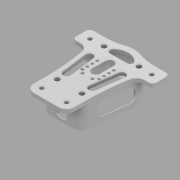
# Autodesk Inventor part: Arm - mounting bottom
Saved by Autodesk Inventor 2017 (Build 210142000, 142)
## iProperties
Created: 2016-04-07
Part Number: Arm - mounting bottom
Material: Generic
Document SubType Name: Modeling
Designer: Ali
Density: 1 g/cm^3
Appearance: Default
Author: Ali
Autodesk Inventor part; units mm, degrees
ref_plane "XZ Plane" through (0, 0, 0) normal (0, 1, 0) x (-1, 0, 0)
sketch "Sketch1" plane through (0, 0, 0) normal (0, 0, 1) x (1, 0, 0)
  circle A0 centre (8.018, -62.9011) radius 2.15 construction
  circle A1 centre (16.3016, 21.0861) radius 2.15 construction
  circle A2 centre (-32.018, -62.9011) radius 2.15 construction
  circle A3 centre (-40.3016, 21.0861) radius 2.15 construction
  arc A4 (-45.0145, -63.2021) -> (-32.018, -75.9011) centre (-32.018, -62.9011) ccw construction
  line L0 (-32.018, -75.9011) -> (8.018, -75.9011) construction
  arc A5 (8.018, -75.9011) -> (21.0145, -63.2021) centre (8.018, -62.9011) ccw projected
  arc A6 (26.6625, -4.5967) -> (21.0145, -63.2021) centre (424.9844, -72.5593) ccw projected
  arc A7 (26.6625, -4.5967) -> (-50.6625, -4.5967) centre (-12, 2) ccw construction
  arc A8 (-45.0145, -63.2021) -> (-50.6625, -4.5967) centre (-448.9844, -72.5593) ccw construction
  circle A9 centre (-12, 2) radius 21 construction
  line L1 (0.5858, -1.5) -> (2.5, -1.5) construction
  line L2 (0.5858, -1.5) -> (0.5858, 0) construction
  line L3 (0.5858, 0) -> (0, 0) construction
  line L4 (0, 0) -> (0, 8.5) construction
  arc A10 (0, 8.5) -> (-4, 12.5) centre (-4, 8.5) ccw construction
  line L5 (-4, 12.5) -> (-20, 12.5) construction
  arc A11 (-20, 12.5) -> (-24, 8.5) centre (-20, 8.5) ccw construction
  line L6 (-24, 8.5) -> (-24, 0) construction
  line L7 (-24.5858, 0) -> (-24, 0) construction
  line L8 (-24.5858, 0) -> (-24.5858, -1.5) construction
  line L9 (-24.5858, -1.5) -> (-26.5, -1.5) construction
  line L10 (-26.5, -1.7) -> (-26.5, -1.5) construction
  line L11 (-26.5, -1.7) -> (-26.9172, -1.7) construction
  line L12 (-26.9172, -1.7) -> (-26.9172, -7.8) construction
  line L13 (-26.9172, -7.8) -> (-24.5858, -7.8) construction
  line L14 (-24.5858, -7.8) -> (-24.5858, -9.7) construction
  line L15 (-24.5858, -9.7) -> (-26.9172, -9.7) construction
  line L16 (-26.9172, -9.7) -> (-26.9172, -15.8) construction
  line L17 (-26.9172, -15.8) -> (-24.5858, -15.8) construction
  line L18 (-24.5858, -15.8) -> (-24.5858, -17.7) construction
  line L19 (-24.5858, -17.7) -> (-26.9172, -17.7) construction
  line L20 (-26.9172, -17.7) -> (-26.9172, -23.8) construction
  line L21 (-26.9172, -23.8) -> (-24.5858, -23.8) construction
  line L22 (-24.5858, -23.8) -> (-24.5858, -25.7) construction
  line L23 (-24.5858, -25.7) -> (-26.9172, -25.7) construction
  line L24 (-26.9172, -25.7) -> (-26.9172, -31.8) construction
  line L25 (-26.9172, -31.8) -> (-25, -31.8) construction
  line L26 (-25, -31.8) -> (-25, -33.5) construction
  line L27 (-23.5, -33.5) -> (-25, -33.5) construction
  line L28 (-23.5, -33.5) -> (-23.5, -35) construction
  line L29 (-23.05, -35) -> (-23.5, -35) construction
  line L30 (-23.05, -35) -> (-23.05, -35.4172) construction
  line L31 (-23.05, -35.4172) -> (-16.95, -35.4172) construction
  line L32 (-16.95, -35.4172) -> (-16.95, -32.9172) construction
  line L33 (-16.95, -32.9172) -> (-7.05, -32.9172) construction
  line L34 (-7.05, -32.9172) -> (-7.05, -35.4172) construction
  line L35 (-7.05, -35.4172) -> (-0.95, -35.4172) construction
  line L36 (-0.95, -35.4172) -> (-0.95, -35) construction
  line L37 (-0.95, -35) -> (-0.5, -35) construction
  line L38 (-0.5, -33.5) -> (-0.5, -35) construction
  line L39 (-0.5, -33.5) -> (1, -33.5) construction
  line L40 (1, -31.8) -> (1, -33.5) construction
  line L41 (1, -31.8) -> (2.9172, -31.8) construction
  line L42 (2.9172, -31.8) -> (2.9172, -25.7) construction
  line L43 (2.9172, -25.7) -> (0.5858, -25.7) construction
  line L44 (0.5858, -25.7) -> (0.5858, -23.8) construction
  line L45 (0.5858, -23.8) -> (2.9172, -23.8) construction
  line L46 (2.9172, -23.8) -> (2.9172, -17.7) construction
  line L47 (2.9172, -17.7) -> (0.5858, -17.7) construction
  line L48 (0.5858, -17.7) -> (0.5858, -15.8) construction
  line L49 (0.5858, -15.8) -> (2.9172, -15.8) construction
  line L50 (2.9172, -15.8) -> (2.9172, -9.7) construction
  line L51 (2.9172, -9.7) -> (0.5858, -9.7) construction
  line L52 (0.5858, -9.7) -> (0.5858, -7.8) construction
  line L53 (0.5858, -7.8) -> (2.9172, -7.8) construction
  line L54 (2.9172, -7.8) -> (2.9172, -1.7) construction
  line L55 (2.9172, -1.7) -> (2.5, -1.7) construction
  line L56 (2.5, -1.7) -> (2.5, -1.5) construction
  line L57 (-26, -2.5) -> (-25, -2.5) construction
  line L58 (-25, -2.5) -> (-25, -3.6044) construction
  arc A12 (-25, -5.8956) -> (-25, -3.6044) centre (-25.5, -4.75) ccw construction
  line L59 (-25, -5.8956) -> (-25, -7) construction
  line L60 (-25, -7) -> (-26, -7) construction
  line L61 (-26, -7) -> (-26, -5.8956) construction
  arc A13 (-26, -3.6044) -> (-26, -5.8956) centre (-25.5, -4.75) ccw construction
  line L62 (-26, -3.6044) -> (-26, -2.5) construction
  line L63 (-26, -10.5) -> (-25, -10.5) construction
  line L64 (-25, -10.5) -> (-25, -11.6044) construction
  arc A14 (-25, -13.8956) -> (-25, -11.6044) centre (-25.5, -12.75) ccw construction
  line L65 (-25, -13.8956) -> (-25, -15) construction
  line L66 (-25, -15) -> (-26, -15) construction
  line L67 (-26, -15) -> (-26, -13.8956) construction
  arc A15 (-26, -11.6044) -> (-26, -13.8956) centre (-25.5, -12.75) ccw construction
  line L68 (-26, -11.6044) -> (-26, -10.5) construction
  line L69 (-26, -18.5) -> (-25, -18.5) construction
  line L70 (-25, -18.5) -> (-25, -19.6044) construction
  arc A16 (-25, -21.8956) -> (-25, -19.6044) centre (-25.5, -20.75) ccw construction
  line L71 (-25, -21.8956) -> (-25, -23) construction
  line L72 (-25, -23) -> (-26, -23) construction
  line L73 (-26, -23) -> (-26, -21.8956) construction
  arc A17 (-26, -19.6044) -> (-26, -21.8956) centre (-25.5, -20.75) ccw construction
  line L74 (-26, -19.6044) -> (-26, -18.5) construction
  line L75 (-26, -26.5) -> (-25, -26.5) construction
  line L76 (-25, -26.5) -> (-25, -27.6044) construction
  arc A18 (-25, -29.8956) -> (-25, -27.6044) centre (-25.5, -28.75) ccw construction
  line L77 (-25, -29.8956) -> (-25, -31.0635) construction
  line L78 (-25, -31.0635) -> (-26, -31.0635) construction
  line L79 (-26, -31.0635) -> (-26, -29.8956) construction
  arc A19 (-26, -27.6044) -> (-26, -29.8956) centre (-25.5, -28.75) ccw construction
  line L80 (-26, -27.6044) -> (-26, -26.5) construction
  line L81 (-2, -8.8) -> (-2, 8.5) construction
  line L82 (-2, -8.8) -> (-1.95, -8.8) construction
  arc A20 (-1.55, -9.2) -> (-1.95, -8.8) centre (-1.95, -9.2) ccw construction
  line L83 (-1.55, -9.2) -> (-1.55, -17.8) construction
  arc A21 (-1.95, -18.2) -> (-1.55, -17.8) centre (-1.95, -17.8) ccw construction
  line L84 (-1.95, -18.2) -> (-2, -18.2) construction
  line L85 (-2, -30.25) -> (-2, -18.2) construction
  arc A22 (-2.25, -30.5) -> (-2, -30.25) centre (-2.25, -30.25) ccw construction
  line L86 (-21.75, -30.5) -> (-2.25, -30.5) construction
  arc A23 (-22, -30.25) -> (-21.75, -30.5) centre (-21.75, -30.25) ccw construction
  line L87 (-22, -18.2) -> (-22, -30.25) construction
  line L88 (-22, -18.2) -> (-22.05, -18.2) construction
  arc A24 (-22.45, -17.8) -> (-22.05, -18.2) centre (-22.05, -17.8) ccw construction
  line L89 (-22.45, -17.8) -> (-22.45, -9.2) construction
  arc A25 (-22.05, -8.8) -> (-22.45, -9.2) centre (-22.05, -9.2) ccw construction
  line L90 (-22.05, -8.8) -> (-22, -8.8) construction
  line L91 (-22, 8.5) -> (-22, -8.8) construction
  arc A26 (-20, 10.5) -> (-22, 8.5) centre (-20, 8.5) ccw construction
  line L92 (-14, 10.5) -> (-20, 10.5) construction
  line L93 (-10, 10.5) -> (-14, 10.5) construction
  line L94 (-4, 10.5) -> (-10, 10.5) construction
  arc A27 (-2, 8.5) -> (-4, 10.5) centre (-4, 8.5) ccw construction
  line L95 (2, -26.5) -> (1, -26.5) construction
  line L96 (2, -27.6044) -> (2, -26.5) construction
  arc A28 (2, -29.8956) -> (2, -27.6044) centre (1.5, -28.75) ccw construction
  line L97 (2, -31.0635) -> (2, -29.8956) construction
  line L98 (1, -31.0635) -> (2, -31.0635) construction
  line L99 (1, -29.8956) -> (1, -31.0635) construction
  arc A29 (1, -27.6044) -> (1, -29.8956) centre (1.5, -28.75) ccw construction
  line L100 (1, -26.5) -> (1, -27.6044) construction
  line L101 (2, -18.5) -> (1, -18.5) construction
  line L102 (2, -19.6044) -> (2, -18.5) construction
  arc A30 (2, -21.8956) -> (2, -19.6044) centre (1.5, -20.75) ccw construction
  line L103 (2, -23) -> (2, -21.8956) construction
  line L104 (1, -23) -> (2, -23) construction
  line L105 (1, -21.8956) -> (1, -23) construction
  arc A31 (1, -19.6044) -> (1, -21.8956) centre (1.5, -20.75) ccw construction
  line L106 (1, -18.5) -> (1, -19.6044) construction
  line L107 (2, -10.5) -> (1, -10.5) construction
  line L108 (2, -11.6044) -> (2, -10.5) construction
  arc A32 (2, -13.8956) -> (2, -11.6044) centre (1.5, -12.75) ccw construction
  line L109 (2, -15) -> (2, -13.8956) construction
  line L110 (1, -15) -> (2, -15) construction
  line L111 (1, -13.8956) -> (1, -15) construction
  arc A33 (1, -11.6044) -> (1, -13.8956) centre (1.5, -12.75) ccw construction
  line L112 (1, -10.5) -> (1, -11.6044) construction
  line L113 (2, -2.5) -> (1, -2.5) construction
  line L114 (2, -3.6044) -> (2, -2.5) construction
  arc A34 (2, -5.8956) -> (2, -3.6044) centre (1.5, -4.75) ccw construction
  line L115 (2, -7) -> (2, -5.8956) construction
  line L116 (1, -7) -> (2, -7) construction
  line L117 (1, -5.8956) -> (1, -7) construction
  arc A35 (1, -3.6044) -> (1, -5.8956) centre (1.5, -4.75) ccw construction
  line L118 (1, -2.5) -> (1, -3.6044) construction
  line L119 (-6.3135, -34.5) -> (-5.1456, -34.5) construction
  line L120 (-6.3135, -33.5) -> (-6.3135, -34.5) construction
  line L121 (-5.1456, -33.5) -> (-6.3135, -33.5) construction
  arc A36 (-2.8544, -33.5) -> (-5.1456, -33.5) centre (-4, -34) ccw construction
  line L122 (-1.6865, -33.5) -> (-2.8544, -33.5) construction
  line L123 (-1.6865, -34.5) -> (-1.6865, -33.5) construction
  line L124 (-2.8544, -34.5) -> (-1.6865, -34.5) construction
  arc A37 (-5.1456, -34.5) -> (-2.8544, -34.5) centre (-4, -34) ccw construction
  line L125 (-17.6865, -33.5) -> (-17.6865, -34.5) construction
  line L126 (-17.6865, -34.5) -> (-18.8544, -34.5) construction
  arc A38 (-21.1456, -34.5) -> (-18.8544, -34.5) centre (-20, -34) ccw construction
  line L127 (-21.1456, -34.5) -> (-22.3135, -34.5) construction
  line L128 (-22.3135, -34.5) -> (-22.3135, -33.5) construction
  line L129 (-22.3135, -33.5) -> (-21.1456, -33.5) construction
  arc A39 (-18.8544, -33.5) -> (-21.1456, -33.5) centre (-20, -34) ccw construction
  line L130 (-18.8544, -33.5) -> (-17.6865, -33.5) construction
  line L131 (-12, -83.0246) -> (-12, 52.1033) construction
  line L132 (-1.5, 12) -> (-12, 12)
  line L133 (-1.5, -31) -> (-12, -31)
  line L134 (-1.5, -31) -> (-1.5, 12)
  line L135 (8.018, -75.9011) -> (-12, -75.9011)
  arc A40 (26.6625, -4.5967) -> (-12, 41.2213) centre (-12, 2) ccw
  arc A41 (-45.0145, -63.2021) -> (-32.018, -75.9011) centre (-32.018, -62.9011) ccw
  arc A42 (-45.0145, -63.2021) -> (-50.6625, -4.5967) centre (-448.9844, -72.5593) ccw
  line L136 (-32.018, -75.9011) -> (-12, -75.9011)
  arc A43 (-12, 41.2213) -> (-50.6625, -4.5967) centre (-12, 2) ccw
  line L137 (-22.5, 12) -> (-12, 12)
  line L138 (-22.5, -31) -> (-12, -31)
  line L139 (-22.5, -31) -> (-22.5, 12)
  dimension "d2" = 21
  dimension "d3" = 10
  dimension "d4" = 33
  constraints: 18 end point, 4 point on circle, 4 point on line, 4 symmetric about line, 2 centre point, 2 perpendicular, 2 vertical, 1 coincident, 1 midpoint, 3 other
  measures "d2" diameter of L134 L131
  measures "d3" distance from line of L132 A7.centre
  measures "d4" distance from line of L133 A7.centre
extrude "Extrusion1" add sketch "Sketch1" along normal blind 5
sketch "Sketch2" plane through (0, 0, 0) normal (0, 0, -1) x (-1, 0, 0)
  line L0 (32.018, -75.9011) -> (-8.018, -75.9011) projected
  arc A0 (32.018, -75.9011) -> (45.0145, -63.2021) centre (32.018, -62.9011) ccw projected
  arc A1 (50.6625, -4.5967) -> (45.0145, -63.2021) centre (448.9844, -72.5593) ccw projected
  arc A2 (50.6625, -4.5967) -> (-26.6625, -4.5967) centre (12, 2) ccw projected
  arc A3 (-21.0145, -63.2021) -> (-26.6625, -4.5967) centre (-424.9844, -72.5593) ccw projected
  arc A4 (-21.0145, -63.2021) -> (-8.018, -75.9011) centre (-8.018, -62.9011) ccw projected
  arc A5 (49.6768, -4.4285) -> (44.0148, -63.179) centre (448.9844, -72.5593) ccw
  line L1 (32.018, -74.9011) -> (-8.018, -74.9011)
  arc A6 (-20.0148, -63.179) -> (-25.6768, -4.4285) centre (-424.9844, -72.5593) ccw
  circle A7 centre (40.3016, 21.0861) radius 2.15 projected
  circle A8 centre (-16.3016, 21.0861) radius 2.15 projected
  circle A9 centre (-8.018, -62.9011) radius 2.15 projected
  circle A10 centre (32.018, -62.9011) radius 2.15 projected
  line L2 (12, 2) -> (40.3016, 21.0861) construction
  line L3 (40.3016, 21.0861) -> (56.7899, 32.2056) construction
  arc A11 (36.9468, 26.0606) -> (43.6563, 16.1116) centre (40.3016, 21.0861) ccw
  line L4 (43.6563, 16.1116) -> (46.6505, 18.1309)
  line L5 (39.9411, 28.0799) -> (36.9468, 26.0606)
  arc A12 (49.6768, -4.4285) -> (46.6505, 18.1309) centre (12, 2) ccw
  line L6 (12, 58.4423) -> (12, -105.8991)
  arc A13 (-19.6563, 16.1116) -> (-12.9468, 26.0606) centre (-16.3016, 21.0861) ccw
  line L7 (-19.6563, 16.1116) -> (-22.6505, 18.1309)
  line L8 (-15.9411, 28.0799) -> (-12.9468, 26.0606)
  arc A14 (39.9411, 28.0799) -> (-15.9411, 28.0799) centre (12, 2) ccw
  arc A15 (-22.6505, 18.1309) -> (-25.6768, -4.4285) centre (12, 2) ccw
  arc A16 (36.8978, -65.7489) -> (34.7521, -67.8455) centre (32.018, -62.9011) ccw
  line L9 (32.018, -62.9011) -> (40.4045, -71.4841) construction
  line L10 (34.7521, -67.8455) -> (39.3316, -72.5324)
  line L11 (36.8978, -65.7489) -> (41.4773, -70.4357)
  arc A17 (32.018, -74.9011) -> (39.2658, -72.465) centre (32.018, -62.9011) ccw
  arc A18 (41.4116, -70.3684) -> (44.0148, -63.179) centre (32.018, -62.9011) ccw
  arc A19 (-10.7521, -67.8455) -> (-12.8978, -65.7489) centre (-8.018, -62.9011) ccw
  line L12 (-10.7521, -67.8455) -> (-15.3316, -72.5324)
  line L13 (-12.8978, -65.7489) -> (-17.4773, -70.4357)
  arc A20 (-20.0148, -63.179) -> (-17.4116, -70.3684) centre (-8.018, -62.9011) ccw
  arc A21 (-15.2658, -72.465) -> (-8.018, -74.9011) centre (-8.018, -62.9011) ccw
  point P0 (0, 0)
  point P1 (48.5457, 26.6459)
  dimension "d9" = 6
  dimension "d10" = 3.5
  dimension "d11" = 1.5
  constraints: 28 end point, 26 point on circle, 13 centre point, 12 symmetric about line, 5 point on line, 2 parallel, 2 tangent, 1 midpoint, 1 vertical, 2 other
  measures "d9" radius of A11
  measures "d10" radial gap between concentric circles of A10 A16
  measures "d11" distance between parallel lines of L9 L10
ref_plane "Work Plane1" through (-51.2213, -75.9011, -38) normal (0, 0, 1) x (1, 0, 0)
extrude "Extrusion2" add sketch "Sketch2" along normal up to surface (38 mm away) contours L0 L6 L1 A17 L10 A16 L11 A18 A5 A12 L4 A11 L5 A14 A2 A1 A0 | L0 A4 A3 A2 L6 A14 L8 A13 L7 A15 A6 A20 L13 A19 L12 A21 L1
sketch "Sketch4" plane through (-32.018, -75.9011, 5) normal (0, -1, 0) x (1, 0, 0)
  line L0 (22.7813, -17.9259) -> (17.2547, -17.9259)
  line L1 (11.2547, -23.9259) -> (11.2547, -32.7215)
  line L2 (17.2547, -38.7215) -> (22.7813, -38.7215)
  line L3 (28.7813, -32.7215) -> (28.7813, -23.9259)
  line L4 (28.7813, -17.9259) -> (11.2547, -38.7215) construction
  line L5 (11.2547, -17.9259) -> (28.7813, -38.7215) construction
  arc A0 (22.7813, -38.7215) -> (28.7813, -32.7215) centre (22.7813, -32.7215) ccw
  arc A1 (11.2547, -32.7215) -> (17.2547, -38.7215) centre (17.2547, -32.7215) ccw
  arc A2 (17.2547, -17.9259) -> (11.2547, -23.9259) centre (17.2547, -23.9259) ccw
  arc A3 (28.7813, -23.9259) -> (22.7813, -17.9259) centre (22.7813, -23.9259) ccw
  point P0 (32.018, -5)
  point P1 (20.018, -28.3237)
  dimension "d16" = 6
  constraints: 12 end point, 8 point on circle, 8 point on line, 8 tangent, 4 centre point, 3 equal radius, 2 midpoint, 2 parallel, 1 horizontal, 1 perpendicular, 1 other
  measures "d16" radius of A0
extrude "Extrusion4" cut sketch "Sketch4" against normal up to next
fillet "Fillet1" radius 2 34 edges at (-46.6505, 18.1309, -19) (-39.9411, 28.0799, -19) (-41.4116, -70.3684, -19) (-36.8978, -65.7489, -19) (-39.2658, -72.465, -19) (-34.7521, -67.8455, -19) (-49.8819, 7.0817, 0) (-43.3011, -66.9866, 0) (-45.7743, -33.7005, 0) (-12, 40.2213, 0) (-38.444, 27.0703, 0) (-45.1534, 17.1212, 0) (-35.3271, 17.7314, 0) (-35.8411, -74.2758, 0) (11.8411, -74.2758, 0) (-12, -74.9011, 0) (19.3011, -66.9866, 0) (25.8819, 7.0817, 0) (21.7743, -33.7005, 0) (4.0694, -58.8599, 0) (10.7521, -67.8455, -19) (15.2658, -72.465, -19) (17.4116, -70.3684, -19) (12.8978, -65.7489, -19) (13.0089, -70.1553, 0) (15.1547, -68.0587, 0) (-39.1547, -68.0587, 0) (-37.0089, -70.1553, 0) (15.9411, 28.0799, -19) (21.1534, 17.1212, 0) (14.444, 27.0703, 0) (11.3271, 17.7314, 0) (22.6505, 18.1309, -19) (-28.0694, -58.8599, 0)
sketch "Sketch7" plane through (0, 0, 0) normal (0, 0, -1) x (-1, 0, 0)
  line L0 (1.5, -31) -> (22.5, -31) projected
  line L1 (16.5002, -31) -> (7.5045, -31)
  line L2 (7.5045, -31) -> (7.5045, -53.6732)
  line L3 (7.5045, -53.6732) -> (16.5002, -53.6732)
  line L4 (16.5002, -53.6732) -> (16.5002, -31)
  point P0 (0, 0)
  constraints: 8 end point, 2 parallel, 1 horizontal, 1 perpendicular, 1 point on line
extrude "Extrusion7" cut sketch "Sketch7" against normal blind 3.5
fillet "Fillet3" radius 6 2 edges at (-12.0024, -53.6732, 3.5) (-12.0024, -53.6732, 0)
sketch "Sketch8" plane through (0, 0, 5) normal (0, 0, 1) x (1, 0, 0)
  line L0 (-1.5, 12) -> (-1.5, -31) projected
  line L1 (-1.5, -31) -> (-22.5, -31) projected
  line L2 (-22.5, -31) -> (-22.5, 12) projected
  line L3 (-22.5, 12) -> (-1.5, 12) projected
  point P0 (0, 0)
extrude "Extrusion8" add sketch "Sketch8" against normal blind 1.5
sketch "Sketch10" plane through (0, 0, 5) normal (0, 0, 1) x (1, 0, 0)
  line L0 (-70.7409, 34.4584) -> (-34.0172, 34.4584)
  line L1 (52.7409, 28.4584) -> (52.7409, 12.5917)
  line L2 (46.7409, 6.5917) -> (26.9516, 6.5917)
  line L3 (-76.7409, 12.5917) -> (-76.7409, 20.525)
  line L4 (-12, 67.6046) -> (-12, -83.4161) construction
  line L5 (10.0172, 34.4584) -> (46.7409, 34.4584)
  line L6 (-123.6927, 20.525) -> (99.0882, 20.525) construction
  line L7 (-76.7409, 20.525) -> (-76.7409, 28.4584)
  arc A0 (46.7409, 6.5917) -> (52.7409, 12.5917) centre (46.7409, 12.5917) ccw
  arc A1 (52.7409, 28.4584) -> (46.7409, 34.4584) centre (46.7409, 28.4584) ccw
  arc A2 (-70.7409, 34.4584) -> (-76.7409, 28.4584) centre (-70.7409, 28.4584) ccw
  arc A3 (-76.7409, 12.5917) -> (-70.7409, 6.5917) centre (-70.7409, 12.5917) ccw
  arc A4 (26.9516, 6.5917) -> (10.0172, 34.4584) centre (-12, 2) ccw
  arc A5 (-34.0172, 34.4584) -> (-50.9516, 6.5917) centre (-12, 2) ccw
  line L8 (-50.9516, 6.5917) -> (-70.7409, 6.5917)
  line L9 (-32.018, -100.9245) -> (-12, -100.9245)
  arc A6 (8.018, -100.9245) -> (21.0145, -88.2255) centre (8.018, -87.9245) ccw
  arc A7 (-45.0145, -88.2255) -> (-32.018, -100.9245) centre (-32.018, -87.9245) ccw
  line L10 (-12, -100.9245) -> (8.018, -100.9245)
  line L11 (21.0145, -88.2255) -> (21.0145, -63.2021)
  arc A8 (8.018, -75.9011) -> (21.0145, -63.2021) centre (8.018, -62.9011) ccw projected
  line L12 (-32.018, -75.9011) -> (8.018, -75.9011) projected
  arc A9 (-45.0145, -63.2021) -> (-32.018, -75.9011) centre (-32.018, -62.9011) ccw projected
  line L13 (-45.0145, -88.2255) -> (-45.0145, -63.2021)
  point P0 (0, 0)
  dimension "d30" = 6
  dimension "d31" = 6
  constraints: 26 end point, 18 point on circle, 10 tangent, 8 centre point, 6 parallel, 4 horizontal, 3 point on line, 3 vertical, 2 collinear, 2 equal radius, 2 perpendicular, 1 other
  measures "d30" radius of A0
  measures "d31" radius of A1
extrude "Extrusion9" add sketch "Sketch10" against normal blind 6
fillet "Fillet4" radius 90 2 edges at (-34.0172, 34.4584, 2) (10.0172, 34.4584, 2)
fillet "Fillet5" radius 13.75 2 edges at (26.9516, 6.5917, 2) (-50.9516, 6.5917, 2)
fillet "Fillet6" radius 3 7 edges at (26.6406, -4.7256, -1) (21.6722, 22.112, -1) (-50.6406, -4.7256, -1) (-45.6722, 22.112, -1) (-41.1033, -72.1993, -1) (17.1033, -72.1993, -1) (-12, -75.9011, -1)
sketch "Sketch11" plane through (0, 0, 5) normal (0, 0, 1) x (1, 0, 0)
  arc A0 (40.1743, 6.5917) -> (26.6186, -4.8545) centre (40.1743, -7.1583) ccw projected
  line L0 (46.7409, 6.5917) -> (40.1743, 6.5917) projected
  arc A1 (46.7409, 6.5917) -> (52.7409, 12.5917) centre (46.7409, 12.5917) ccw projected
  line L1 (52.7409, 28.4584) -> (52.7409, 12.5917) projected
  arc A2 (52.7409, 28.4584) -> (46.7409, 34.4584) centre (46.7409, 28.4584) ccw projected
  line L2 (29.2562, 34.4584) -> (46.7409, 34.4584) projected
  arc A3 (0.5221, 39.1686) -> (29.2562, 34.4584) centre (29.2562, 124.4584) ccw projected
  arc A4 (0.5221, 39.1686) -> (-24.5221, 39.1686) centre (-12, 2) ccw projected
  arc A5 (-53.2562, 34.4584) -> (-24.5221, 39.1686) centre (-53.2562, 124.4584) ccw projected
  line L3 (-53.2562, 34.4584) -> (-70.7409, 34.4584) projected
  arc A6 (-70.7409, 34.4584) -> (-76.7409, 28.4584) centre (-70.7409, 28.4584) ccw projected
  line L4 (-76.7409, 28.4584) -> (-76.7409, 12.5917) projected
  arc A7 (-76.7409, 12.5917) -> (-70.7409, 6.5917) centre (-70.7409, 12.5917) ccw projected
  line L5 (-70.7409, 6.5917) -> (-64.1743, 6.5917) projected
  arc A8 (-50.6186, -4.8545) -> (-64.1743, 6.5917) centre (-64.1743, -7.1583) ccw projected
  arc A9 (-45.0145, -63.2021) -> (-50.6186, -4.8545) centre (-448.9844, -72.5593) ccw projected
  line L6 (-45.0145, -63.2021) -> (-45.0145, -88.2255) projected
  arc A10 (-45.0145, -88.2255) -> (-32.018, -100.9245) centre (-32.018, -87.9245) ccw projected
  line L7 (-32.018, -100.9245) -> (8.018, -100.9245) projected
  arc A11 (8.018, -100.9245) -> (21.0145, -88.2255) centre (8.018, -87.9245) ccw projected
  line L8 (21.0145, -88.2255) -> (21.0145, -63.2021) projected
  arc A12 (26.6186, -4.8545) -> (21.0145, -63.2021) centre (424.9844, -72.5593) ccw projected
  line L9 (-12, 2) -> (-12, 28.4584)
  point P0 (0, 0)
  point P1 (38, 20.0755)
  point P2 (-62, 20.0755)
  point P3 (-32.018, -87.9245)
  dimension "d44" = 100
  dimension "d45" = 108
  constraints: 2 end point, 2 symmetric about line, 1 coincident, 1 vertical
  measures "d44" distance of point (-62, 20.076) point (38, 20.076)
  measures "d45" vertical distance of point (-62, 20.076) point (-32.018, -87.924)
hole "Hole1" at (38, 20.0755, 5) at (8.018, -87.9245, 5) at (-62, 20.0755, 5) at (-32.018, -87.9245, 5) direction (0, 0, -1) diameter 6.5 end through all
sketch "Sketch12" plane through (0, 0, 5) normal (0, 0, 1) x (1, 0, 0)
  circle A0 centre (8.018, -62.9011) radius 2.15 projected
  circle A1 centre (-32.018, -62.9011) radius 2.15 projected
  circle A2 centre (-40.3016, 21.0861) radius 2.15 projected
  circle A3 centre (16.3016, 21.0861) radius 2.15 projected
  point P0 (0, 0)
hole "Hole2" at (-32.018, -62.9011, 5) at (8.018, -62.9011, 5) at (-40.3016, 21.0861, 5) at (16.3016, 21.0861, 5) direction (0, 0, -1) diameter 4.5 end through all counterbore diameter 8 counterbore depth 10
chamfer "Chamfer1" distance 1.75 angle 45 4 edges at (-32.018, -60.6511, -5) (-40.3016, 23.3361, -5) (16.3016, 23.3361, -5) (8.018, -60.6511, -5)
sketch "Sketch13" plane through (0, 0, 5) normal (0, 0, 1) x (1, 0, 0)
  line L0 (0.5858, 0) -> (0, 0) projected
  line L1 (0.5858, 0) -> (0.5858, -1.5) projected
  line L2 (0.5858, -1.5) -> (2.5, -1.5) projected
  line L3 (2.5, -1.7) -> (2.5, -1.5) projected
  line L4 (2.5, -1.7) -> (2.9172, -1.7) projected
  line L5 (2.9172, -1.7) -> (2.9172, -7.8) projected
  line L6 (2.9172, -7.8) -> (0.5858, -7.8) projected
  line L7 (0.5858, -7.8) -> (0.5858, -9.7) projected
  line L8 (0.5858, -9.7) -> (2.9172, -9.7) projected
  line L9 (2.9172, -9.7) -> (2.9172, -15.8) projected
  line L10 (2.9172, -15.8) -> (0.5858, -15.8) projected
  line L11 (0.5858, -15.8) -> (0.5858, -17.7) projected
  line L12 (0.5858, -17.7) -> (2.9172, -17.7) projected
  line L13 (2.9172, -17.7) -> (2.9172, -23.8) projected
  line L14 (2.9172, -23.8) -> (0.5858, -23.8) projected
  line L15 (0.5858, -23.8) -> (0.5858, -25.7) projected
  line L16 (0.5858, -25.7) -> (2.9172, -25.7) projected
  line L17 (2.9172, -25.7) -> (2.9172, -31.8) projected
  line L18 (2.9172, -31.8) -> (1, -31.8) projected
  line L19 (1, -31.8) -> (1, -33.5) projected
  line L20 (-0.5, -33.5) -> (1, -33.5) projected
  line L21 (-0.5, -33.5) -> (-0.5, -35) projected
  line L22 (-0.95, -35) -> (-0.5, -35) projected
  line L23 (-0.95, -35) -> (-0.95, -35.4172) projected
  line L24 (-0.95, -35.4172) -> (-7.05, -35.4172) projected
  line L25 (-7.05, -35.4172) -> (-7.05, -32.9172) projected
  line L26 (-7.05, -32.9172) -> (-16.95, -32.9172) projected
  line L27 (-16.95, -32.9172) -> (-16.95, -35.4172) projected
  line L28 (-16.95, -35.4172) -> (-23.05, -35.4172) projected
  line L29 (-23.05, -35.4172) -> (-23.05, -35) projected
  line L30 (-23.05, -35) -> (-23.5, -35) projected
  line L31 (-23.5, -33.5) -> (-23.5, -35) projected
  line L32 (-23.5, -33.5) -> (-25, -33.5) projected
  line L33 (-25, -31.8) -> (-25, -33.5) projected
  line L34 (-25, -31.8) -> (-26.9172, -31.8) projected
  line L35 (-26.9172, -31.8) -> (-26.9172, -25.7) projected
  line L36 (-26.9172, -25.7) -> (-24.5858, -25.7) projected
  line L37 (-24.5858, -25.7) -> (-24.5858, -23.8) projected
  line L38 (-24.5858, -23.8) -> (-26.9172, -23.8) projected
  line L39 (-26.9172, -23.8) -> (-26.9172, -17.7) projected
  line L40 (-26.9172, -17.7) -> (-24.5858, -17.7) projected
  line L41 (-24.5858, -17.7) -> (-24.5858, -15.8) projected
  line L42 (-24.5858, -15.8) -> (-26.9172, -15.8) projected
  line L43 (-26.9172, -15.8) -> (-26.9172, -9.7) projected
  line L44 (-26.9172, -9.7) -> (-24.5858, -9.7) projected
  line L45 (-24.5858, -9.7) -> (-24.5858, -7.8) projected
  line L46 (-24.5858, -7.8) -> (-26.9172, -7.8) projected
  line L47 (-26.9172, -7.8) -> (-26.9172, -1.7) projected
  line L48 (-26.9172, -1.7) -> (-26.5, -1.7) projected
  line L49 (-26.5, -1.7) -> (-26.5, -1.5) projected
  line L50 (-24.5858, -1.5) -> (-26.5, -1.5) projected
  line L51 (-24.5858, -1.5) -> (-24.5858, 0) projected
  line L52 (-24.5858, 0) -> (-24, 0) projected
  line L53 (-24, 0) -> (-24, 8.25) projected
  line L54 (-24, 8.25) -> (-22, 8.25) projected
  line L55 (-22, -27.25) -> (-22, 8.25) projected
  arc A0 (-22, -27.25) -> (-21.9959, -27.2951) centre (-21.75, -27.25) ccw projected
  arc A1 (-21.9959, -27.2951) -> (-18.7951, -30.4959) centre (-21.5, -30) ccw projected
  arc A2 (-18.7951, -30.4959) -> (-18.75, -30.5) centre (-18.75, -30.25) ccw projected
  line L56 (-5.25, -30.5) -> (-18.75, -30.5) projected
  arc A3 (-5.25, -30.5) -> (-5.2049, -30.4959) centre (-5.25, -30.25) ccw projected
  arc A4 (-5.2049, -30.4959) -> (-2.0041, -27.2951) centre (-2.5, -30) ccw projected
  arc A5 (-2.0041, -27.2951) -> (-2, -27.25) centre (-2.25, -27.25) ccw projected
  line L57 (-2, 8.25) -> (-2, -27.25) projected
  line L58 (-2, 8.25) -> (0, 8.25) projected
  line L59 (0, 8.25) -> (0, 0) projected
  line L60 (2, -2.5) -> (1, -2.5) projected
  line L61 (1, -2.5) -> (1, -3.6044) projected
  arc A6 (1, -3.6044) -> (1, -5.8956) centre (1.5, -4.75) ccw projected
  line L62 (1, -5.8956) -> (1, -7) projected
  line L63 (1, -7) -> (2, -7) projected
  line L64 (2, -7) -> (2, -5.8956) projected
  arc A7 (2, -5.8956) -> (2, -3.6044) centre (1.5, -4.75) ccw projected
  line L65 (2, -3.6044) -> (2, -2.5) projected
  line L66 (2, -10.5) -> (1, -10.5) projected
  line L67 (1, -10.5) -> (1, -11.6044) projected
  arc A8 (1, -11.6044) -> (1, -13.8956) centre (1.5, -12.75) ccw projected
  line L68 (1, -13.8956) -> (1, -15) projected
  line L69 (1, -15) -> (2, -15) projected
  line L70 (2, -15) -> (2, -13.8956) projected
  arc A9 (2, -13.8956) -> (2, -11.6044) centre (1.5, -12.75) ccw projected
  line L71 (2, -11.6044) -> (2, -10.5) projected
  line L72 (2, -18.5) -> (1, -18.5) projected
  line L73 (1, -18.5) -> (1, -19.6044) projected
  arc A10 (1, -19.6044) -> (1, -21.8956) centre (1.5, -20.75) ccw projected
  line L74 (1, -21.8956) -> (1, -23) projected
  line L75 (1, -23) -> (2, -23) projected
  line L76 (2, -23) -> (2, -21.8956) projected
  arc A11 (2, -21.8956) -> (2, -19.6044) centre (1.5, -20.75) ccw projected
  line L77 (2, -19.6044) -> (2, -18.5) projected
  line L78 (2, -26.5) -> (1, -26.5) projected
  line L79 (1, -26.5) -> (1, -27.6044) projected
  arc A12 (1, -27.6044) -> (1, -29.8956) centre (1.5, -28.75) ccw projected
  line L80 (1, -29.8956) -> (1, -31.0635) projected
  line L81 (1, -31.0635) -> (2, -31.0635) projected
  line L82 (2, -31.0635) -> (2, -29.8956) projected
  arc A13 (2, -29.8956) -> (2, -27.6044) centre (1.5, -28.75) ccw projected
  line L83 (2, -27.6044) -> (2, -26.5) projected
  line L84 (-26, -18.5) -> (-25, -18.5) projected
  line L85 (-26, -19.6044) -> (-26, -18.5) projected
  arc A14 (-26, -19.6044) -> (-26, -21.8956) centre (-25.5, -20.75) ccw projected
  line L86 (-26, -23) -> (-26, -21.8956) projected
  line L87 (-25, -23) -> (-26, -23) projected
  line L88 (-25, -21.8956) -> (-25, -23) projected
  arc A15 (-25, -21.8956) -> (-25, -19.6044) centre (-25.5, -20.75) ccw projected
  line L89 (-25, -18.5) -> (-25, -19.6044) projected
  line L90 (-26, -10.5) -> (-25, -10.5) projected
  line L91 (-26, -11.6044) -> (-26, -10.5) projected
  arc A16 (-26, -11.6044) -> (-26, -13.8956) centre (-25.5, -12.75) ccw projected
  line L92 (-26, -15) -> (-26, -13.8956) projected
  line L93 (-25, -15) -> (-26, -15) projected
  line L94 (-25, -13.8956) -> (-25, -15) projected
  arc A17 (-25, -13.8956) -> (-25, -11.6044) centre (-25.5, -12.75) ccw projected
  line L95 (-25, -10.5) -> (-25, -11.6044) projected
  line L96 (-26, -2.5) -> (-25, -2.5) projected
  line L97 (-26, -3.6044) -> (-26, -2.5) projected
  arc A18 (-26, -3.6044) -> (-26, -5.8956) centre (-25.5, -4.75) ccw projected
  line L98 (-26, -7) -> (-26, -5.8956) projected
  line L99 (-25, -7) -> (-26, -7) projected
  line L100 (-25, -5.8956) -> (-25, -7) projected
  arc A19 (-25, -5.8956) -> (-25, -3.6044) centre (-25.5, -4.75) ccw projected
  line L101 (-25, -2.5) -> (-25, -3.6044) projected
  line L102 (-26, -26.5) -> (-25, -26.5) projected
  line L103 (-26, -27.6044) -> (-26, -26.5) projected
  arc A20 (-26, -27.6044) -> (-26, -29.8956) centre (-25.5, -28.75) ccw projected
  line L104 (-26, -31.0635) -> (-26, -29.8956) projected
  line L105 (-25, -31.0635) -> (-26, -31.0635) projected
  line L106 (-25, -29.8956) -> (-25, -31.0635) projected
  arc A21 (-25, -29.8956) -> (-25, -27.6044) centre (-25.5, -28.75) ccw projected
  line L107 (-25, -26.5) -> (-25, -27.6044) projected
  line L108 (-17.6865, -34.5) -> (-18.8544, -34.5) projected
  line L109 (-17.6865, -33.5) -> (-17.6865, -34.5) projected
  line L110 (-18.8544, -33.5) -> (-17.6865, -33.5) projected
  arc A22 (-18.8544, -33.5) -> (-21.1456, -33.5) centre (-20, -34) ccw projected
  line L111 (-22.3135, -33.5) -> (-21.1456, -33.5) projected
  line L112 (-22.3135, -34.5) -> (-22.3135, -33.5) projected
  line L113 (-21.1456, -34.5) -> (-22.3135, -34.5) projected
  arc A23 (-21.1456, -34.5) -> (-18.8544, -34.5) centre (-20, -34) ccw projected
  line L114 (-6.3135, -33.5) -> (-6.3135, -34.5) projected
  line L115 (-6.3135, -34.5) -> (-5.1456, -34.5) projected
  arc A24 (-5.1456, -34.5) -> (-2.8544, -34.5) centre (-4, -34) ccw projected
  line L116 (-2.8544, -34.5) -> (-1.6865, -34.5) projected
  line L117 (-1.6865, -34.5) -> (-1.6865, -33.5) projected
  line L118 (-1.6865, -33.5) -> (-2.8544, -33.5) projected
  arc A25 (-2.8544, -33.5) -> (-5.1456, -33.5) centre (-4, -34) ccw projected
  line L119 (-5.1456, -33.5) -> (-6.3135, -33.5) projected
hole "Hole3" at (-4, -34, 5) at (-20, -34, 5) at (-25.5, -28.75, 5) at (-25.5, -20.75, 5) at (-25.5, -12.75, 5) at (-25.5, -4.75, 5) at (1.5, -28.75, 5) at (1.5, -20.75, 5) at (1.5, -12.75, 5) at (1.5, -4.75, 5) direction (0, 0, -1) diameter 2.5 end through all counterbore diameter 4.5 counterbore depth 2.2
chamfer "Chamfer2" distance 1 angle 45 10 edges at (-4, -32.75, 2.8) (1.5, -27.5, 2.8) (1.5, -19.5, 2.8) (1.5, -11.5, 2.8) (1.5, -3.5, 2.8) (-20, -32.75, 2.8) (-25.5, -27.5, 2.8) (-25.5, -19.5, 2.8) (-25.5, -11.5, 2.8) (-25.5, -3.5, 2.8)
ref_plane "Work Plane4" through (-60, 0, 0) normal (-1, 0, 0) x (0, -1, 0)
sketch "Sketch16" plane through (-12, 2, -38) normal (0, 0, -1) x (-1, 0, 0)
  arc A0 (-33.0145, -65.2021) -> (-20.018, -77.9011) centre (-20.018, -64.9011) ccw projected
  arc A1 (-33.0145, -65.2021) -> (-38.6625, -6.5967) centre (-436.9844, -74.5593) ccw projected
  arc A2 (38.6625, -6.5967) -> (-38.6625, -6.5967) centre (0, 0) ccw projected
  arc A3 (38.6625, -6.5967) -> (33.0145, -65.2021) centre (436.9844, -74.5593) ccw projected
  arc A4 (20.018, -77.9011) -> (33.0145, -65.2021) centre (20.018, -64.9011) ccw projected
  line L0 (-20.018, -77.9011) -> (20.018, -77.9011) projected
  arc A5 (-29.0156, -65.1095) -> (-20.018, -73.9011) centre (-20.018, -64.9011) ccw
  arc A6 (-29.0156, -65.1095) -> (-34.7195, -5.9239) centre (-436.9844, -74.5593) ccw
  arc A7 (34.7195, -5.9239) -> (-34.7195, -5.9239) centre (0, 0) ccw
  arc A8 (34.7195, -5.9239) -> (29.0156, -65.1095) centre (436.9844, -74.5593) ccw
  arc A9 (20.018, -73.9011) -> (29.0156, -65.1095) centre (20.018, -64.9011) ccw
  line L1 (20.018, -73.9011) -> (-20.018, -73.9011)
  point P0 (-12, -2)
  dimension "d69" = 4
  constraints: 10 point on circle, 5 centre point, 2 end point, 5 other
  measures "d69" radial gap between concentric circles of A0 A5
extrude "Extrusion10" add sketch "Sketch16" against normal blind 3
chamfer "Chamfer3" distance 3 angle 45 10 edges at (-12, 37.2213, -35) (-46.9395, 6.4461, -35) (-42.7881, -33.4127, -35) (-40.543, -65.7863, -35) (22.9395, 6.4461, -35) (18.7881, -33.4127, -35) (16.543, -65.7863, -35) (-12, -71.9011, -35) (-34.7051, -71.4906, -35) (10.7051, -71.4906, -35)
sketch "Sketch17" plane through (0, 0, 0) normal (0, 0, -1) x (-1, 0, 0)
  circle A0 centre (-1.5, -12.75) radius 1.25 projected
  circle A1 centre (-1.5, -28.75) radius 1.25 projected
  circle A2 centre (25.5, -12.75) radius 1.25 projected
  circle A3 centre (25.5, -28.75) radius 1.25 projected
  circle A4 centre (4, -34) radius 1.25 projected
  circle A5 centre (20, -34) radius 1.25 projected
  circle A6 centre (25.5, -20.75) radius 1.25 projected
  circle A7 centre (25.5, -4.75) radius 1.25 projected
  circle A8 centre (-1.5, -20.75) radius 1.25 projected
  circle A9 centre (-1.5, -4.75) radius 1.25 projected
  line L0 (7.5045, -56.6894) -> (7.5045, -31) projected
  line L1 (7.5045, -31) -> (1.5, -31) projected
  line L2 (1.5, -31) -> (1.5, 12) projected
  line L3 (1.5, 12) -> (22.5, 12) projected
  line L4 (22.5, 12) -> (22.5, -31) projected
  line L5 (22.5, -31) -> (16.5002, -31) projected
  line L6 (16.5002, -56.6894) -> (16.5002, -31) projected
  line L7 (7.5045, -56.6894) -> (16.5002, -56.6894) projected
  arc A10 (-12.0613, -72.0472) -> (-8.018, -72.9011) centre (-8.018, -62.9011) ccw projected
  line L8 (32.018, -72.9011) -> (-8.018, -72.9011) projected
  arc A11 (32.018, -72.9011) -> (36.0613, -72.0472) centre (32.018, -62.9011) ccw projected
  line L9 (34.2686, -70.2125) -> (36.0613, -72.0472) projected
  arc A12 (39.2754, -65.3204) -> (34.2686, -70.2125) centre (32.018, -62.9011) ccw projected
  line L10 (41.068, -67.1551) -> (39.2754, -65.3204) projected
  arc A13 (41.068, -67.1551) -> (42.0153, -63.1327) centre (32.018, -62.9011) ccw projected
  arc A14 (47.7053, -4.0921) -> (42.0153, -63.1327) centre (448.9844, -72.5593) ccw projected
  arc A15 (47.7053, -4.0921) -> (45.7619, 15.1193) centre (12, 2) ccw projected
  line L11 (44.7745, 14.4534) -> (45.7619, 15.1193) projected
  arc A16 (35.8286, 27.7188) -> (44.7745, 14.4534) centre (40.3016, 21.0861) ccw projected
  line L12 (36.8159, 28.3847) -> (35.8286, 27.7188) projected
  arc A17 (36.8159, 28.3847) -> (-12.8159, 28.3847) centre (12, 2) ccw projected
  line L13 (-11.8286, 27.7188) -> (-12.8159, 28.3847) projected
  arc A18 (-20.7745, 14.4534) -> (-11.8286, 27.7188) centre (-16.3016, 21.0861) ccw projected
  line L14 (-21.7619, 15.1193) -> (-20.7745, 14.4534) projected
  arc A19 (-21.7619, 15.1193) -> (-23.7053, -4.0921) centre (12, 2) ccw projected
  arc A20 (-18.0153, -63.1327) -> (-23.7053, -4.0921) centre (-424.9844, -72.5593) ccw projected
  arc A21 (-18.0153, -63.1327) -> (-17.068, -67.1551) centre (-8.018, -62.9011) ccw projected
  line L15 (-15.2754, -65.3204) -> (-17.068, -67.1551) projected
  arc A22 (-10.2686, -70.2125) -> (-15.2754, -65.3204) centre (-8.018, -62.9011) ccw projected
  line L16 (-12.0613, -72.0472) -> (-10.2686, -70.2125) projected
  line L17 (32.5187, -46.656) -> (38.2234, -4.6893) construction
  line L18 (38.4217, -47.4584) -> (44.1264, -5.4917)
  line L19 (32.3204, -3.8868) -> (26.6157, -45.8536)
  arc A23 (26.6157, -45.8536) -> (38.4217, -47.4584) centre (32.5187, -46.656) ccw
  arc A24 (44.1264, -5.4917) -> (32.3204, -3.8868) centre (38.2234, -4.6893) ccw
  line L20 (25.8821, 21.0861) -> (-1.8821, 21.0861) construction
  line L21 (25.8821, 16.1256) -> (-1.8821, 16.1256)
  arc A25 (25.8821, 16.1256) -> (29.4681, 24.5136) centre (25.8821, 21.0861) ccw
  arc A26 (-5.4681, 24.5136) -> (-1.8821, 16.1256) centre (-1.8821, 21.0861) ccw
  line L22 (32.018, -71.9011) -> (-8.018, -71.9011) projected
  line L23 (12, -71.9011) -> (12, 37.2213)
  arc A27 (37.4199, 26.3796) -> (-13.4199, 26.3796) centre (12, 2) ccw projected
  line L24 (-8.5187, -46.656) -> (-14.2234, -4.6893) construction
  line L25 (-14.4217, -47.4584) -> (-20.1264, -5.4917)
  line L26 (-8.3204, -3.8868) -> (-2.6157, -45.8536)
  arc A28 (-14.4217, -47.4584) -> (-2.6157, -45.8536) centre (-8.5187, -46.656) ccw
  arc A29 (-8.3204, -3.8868) -> (-20.1264, -5.4917) centre (-14.2234, -4.6893) ccw
  arc A30 (29.4681, 24.5136) -> (-5.4681, 24.5136) centre (12, 7.8176) ccw
  point P0 (0, 0)
  point P1 (35.3711, -25.6726)
  point P2 (12, 21.0861)
  point P3 (-11.3711, -25.6726)
  constraints: 24 end point, 15 point on circle, 8 tangent, 7 centre point, 7 symmetric about line, 3 midpoint, 2 point on line, 1 horizontal, 1 parallel, 2 other
extrude "Extrusion11" cut sketch "Sketch17" against normal through all contours A23 L19 A24 L18 | L21 L23 A30 A25 | L21 A26 A30 L23 | L25 A29 L26 A28
sketch "Sketch18" plane through (0, 0, 5) normal (0, 0, 1) x (1, 0, 0)
  circle A0 centre (16.3016, 21.0861) radius 2.25 projected
  circle A1 centre (-40.3016, 21.0861) radius 2.25 projected
  point P0 (0, 0)
  constraints: 2 coincident
hole "Hole4" at (16.3016, 21.0861, 5) at (-40.3016, 21.0861, 5) direction (0, 0, -1) diameter 4.5 end through all
sketch "Sketch19" plane through (0, 0, 3.5) normal (0, 0, -1) x (-1, 0, 0)
  line L0 (16.5002, -48.2188) -> (7.5045, -48.2188) projected
  line L1 (16.5002, -31) -> (16.5002, -48.2188) projected
  line L2 (22.5, -31) -> (16.5002, -31) projected
  line L3 (22.5, 12) -> (22.5, -31) projected
  line L4 (1.5, 12) -> (22.5, 12) projected
  line L5 (1.5, -31) -> (1.5, 12) projected
  line L6 (7.5045, -31) -> (1.5, -31) projected
  line L7 (7.5045, -48.2188) -> (7.5045, -31) projected
  line L8 (12, -20.0605) -> (12, 1.8137) construction
  line L9 (5.0791, -20.0605) -> (5.0791, 1.8137)
  line L10 (18.9209, 1.8137) -> (18.9209, -20.0605)
  arc A0 (5.0791, -20.0605) -> (18.9209, -20.0605) centre (12, -20.0605) ccw
  arc A1 (18.9209, 1.8137) -> (5.0791, 1.8137) centre (12, 1.8137) ccw
  line L11 (1.5, 12) -> (22.5, 12) projected
  point P0 (0, 0)
  point P1 (12, -9.1234)
  point P2 (12, 12)
  constraints: 8 end point, 4 point on circle, 4 tangent, 2 centre point, 2 midpoint, 1 parallel, 1 point on line, 1 vertical
extrude "Extrusion12" cut sketch "Sketch19" against normal through all contours L9 A1 L10 A0
sketch "Sketch20" plane through (0, 0, 0) normal (1, 0, 0) x (0, 1, 0)
  line L0 (-41.3399, -18.5174) -> (-5.8947, -18.5174) construction
  line L1 (-41.3399, -7.0893) -> (-5.8947, -7.0893)
  line L2 (-5.8947, -29.9456) -> (-41.3399, -29.9456)
  arc A0 (-41.3399, -7.0893) -> (-41.3399, -29.9456) centre (-41.3399, -18.5174) ccw
  arc A1 (-5.8947, -29.9456) -> (-5.8947, -7.0893) centre (-5.8947, -18.5174) ccw
  point P0 (0, 0)
  point P1 (-23.6173, -18.5174)
  constraints: 8 end point, 4 point on circle, 4 tangent, 2 centre point, 1 horizontal, 1 midpoint, 1 parallel
extrude "Extrusion13" cut sketch "Sketch20" along normal through all both and the other way through all
body "Solid1"
